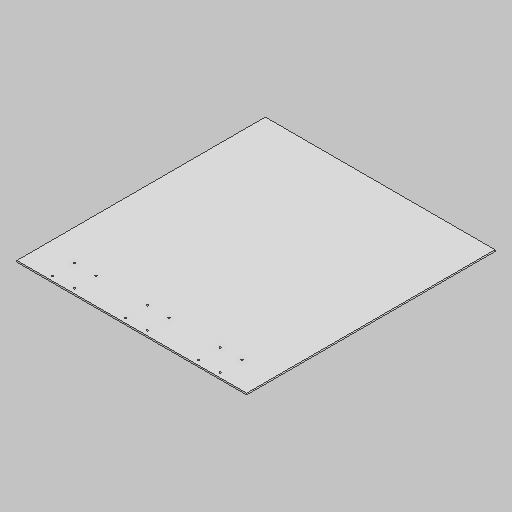
# Autodesk Inventor part: plate2
Saved by Autodesk Inventor 2026.2 (Build 302298000, 298)
## iProperties
Created: 2026-08-10
Part Number: plate2
Material: 일반
Document SubType Name: Modeling
Designer: mjbhang
Density: 1 g/cm^3
Appearance: 기본값
Author: mjbhang
Autodesk Inventor part; units mm, degrees
ref_plane "YZ Plane" through (0, 0, 0) normal (1, 0, 0) x (0, 1, 0)
ref_plane "XZ Plane" through (0, 0, 0) normal (0, 1, 0) x (-1, 0, 0)
ref_plane "XY Plane" through (0, 0, 0) normal (0, 0, 1) x (1, 0, 0)
sketch "스케치1" plane through (0, 0, 0) normal (0, 1, 0) x (-1, 0, 0)
  line L0 (370, -400) -> (-370, -400)
  line L1 (-370, -400) -> (-370, 400)
  line L2 (-370, 400) -> (370, 400)
  line L3 (370, 400) -> (370, -400)
  point P0 (0, 0)
  dimension "d0" = 800
  dimension "d1" = 740
  dimension "d2" = 370
  dimension "d3" = 400
  constraints: 8 end point, 2 parallel, 1 horizontal, 1 perpendicular
  measures "d0" distance of L0.end L1.end
  measures "d1" distance of L0.start L0.end
  measures "d2" distance from line of L1 point (0, 0)
  measures "d3" distance from line of L0 point (0, 0)
extrude "돌출1" add sketch "스케치1" along normal blind 5
sketch "스케치2" plane through (0, 5, 0) normal (0, 1, 0) x (1, 0, 0)
  line L0 (-370, -400) -> (370, -400) projected
  point P0 (0, 0)
  point P1 (-35, -385)
  point P2 (35, -385)
  point P3 (35, -315)
  point P4 (-35, -315)
  dimension "d6" = 15
  dimension "d7" = 15
  dimension "d8" = 35
  dimension "d9" = 35
  dimension "d10" = 35
  dimension "d11" = 35
  dimension "d12" = 70
  dimension "d13" = 70
  measures "d6" distance from line of L0 point (-35, -385)
  measures "d7" distance from line of L0 point (35, -385)
  measures "d8" horizontal distance of point (0, 0) point (-35, -385)
  measures "d9" horizontal distance of point (0, 0) point (35, -385)
  measures "d10" horizontal distance of point (0, 0) point (-35, -315)
  measures "d11" horizontal distance of point (0, 0) point (35, -315)
  measures "d12" distance of point (35, -385) point (35, -315)
  measures "d13" distance of point (-35, -385) point (-35, -315)
hole "구멍1" at (-35, 5, 385) at (35, 5, 385) at (35, 5, 315) at (-35, 5, 315) direction (0, -1, 0) diameter 6 depth 8
sketch "스케치3" plane through (0, 5, 0) normal (0, 1, 0) x (1, 0, 0)
  line L0 (-370, 400) -> (-370, -400) projected
  line L1 (-370, -400) -> (370, -400) projected
  line L2 (370, -400) -> (370, 400) projected
  point P0 (0, 0)
  point P1 (-270, -385)
  point P2 (-200, -385)
  point P3 (-200, -315)
  point P4 (-270, -315)
  point P5 (200, -315)
  point P6 (200, -385)
  point P7 (270, -385)
  point P8 (270, -315)
  dimension "d21" = 100
  dimension "d22" = 100
  dimension "d23" = 70
  dimension "d24" = 15
  dimension "d25" = 15
  dimension "d26" = 70
  dimension "d27" = 70
  dimension "d28" = 70
  dimension "d29" = 100
  dimension "d30" = 100
  dimension "d31" = 15
  dimension "d32" = 15
  dimension "d33" = 70
  dimension "d34" = 70
  dimension "d35" = 70
  measures "d21" distance from line of L0 point (-270, -385)
  measures "d22" distance from line of L0 point (-270, -315)
  measures "d23" distance of point (-270, -385) point (-270, -315)
  measures "d24" distance from line of L1 point (-270, -385)
  measures "d25" distance from line of L1 point (-200, -385)
  measures "d26" distance of point (-200, -385) point (-270, -385)
  measures "d27" distance of point (-200, -315) point (-270, -315)
  measures "d28" distance of point (-200, -385) point (-200, -315)
  measures "d29" distance from line of L2 point (270, -315)
  measures "d30" distance from line of L2 point (270, -385)
  measures "d31" distance from line of L1 point (270, -385)
  measures "d32" distance from line of L1 point (200, -385)
  measures "d33" distance of point (270, -385) point (200, -385)
  measures "d34" distance of point (270, -315) point (200, -315)
  measures "d35" distance of point (270, -385) point (270, -315)
hole "구멍2" at (-270, 5, 385) at (-200, 5, 385) at (-200, 5, 315) at (-270, 5, 315) at (200, 5, 315) at (200, 5, 385) at (270, 5, 385) at (270, 5, 315) direction (0, -1, 0) diameter 6 depth 8
